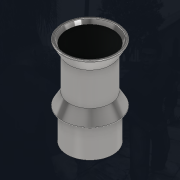
# Autodesk Inventor part: emitter
Saved by Autodesk Inventor 2021 (Build 250183000, 183)
## iProperties
Created: 2021-01-08
Part Number: emitter
Material: Generic
Document SubType Name: Modeling
Designer: Alex
Density: 1 g/cm^3
Appearance: Default
Author: Alex
Autodesk Inventor part; units mm, degrees
ref_plane "YZ Plane" through (0, 0, 0) normal (1, 0, 0) x (0, 1, 0)
ref_plane "XZ Plane" through (0, 0, 0) normal (0, 1, 0) x (-1, 0, 0)
ref_plane "XY Plane" through (0, 0, 0) normal (0, 0, 1) x (1, 0, 0)
sketch "Sketch1" plane through (0, 0, 0) normal (0, 0, 1) x (1, 0, 0)
  line L0 (0, 85.0385) -> (0, 91.0385)
  line L1 (-9, 91.0385) -> (-10, 91.0385)
  line L2 (0, 61.1) -> (0, 78.9)
  line L3 (0, 91.0385) -> (0, 96.0385)
  line L4 (-10, 91.0385) -> (-11, 91.0385)
  line L5 (-9, 91.0385) -> (-9, 85.0385)
  line L6 (-11, 91.0385) -> (-8.1132, 96.0385)
  line L7 (0, 96.0385) -> (0, 109.0385)
  line L8 (0, 96.0385) -> (0, 102.5385) construction
  line L9 (0, 102.5385) -> (-10.5, 102.5385) construction
  line L10 (-11, 114.0385) -> (-8.1132, 109.0385)
  line L11 (0, 114.0385) -> (-8, 114.0385)
  line L12 (-10, 114.0385) -> (-11, 114.0385)
  line L13 (0, 114.0385) -> (-10, 114.0385)
  line L14 (0, 109.0385) -> (0, 114.0385)
  line L15 (-8.1132, 96.0385) -> (-8.1132, 109.0385)
  line L16 (0, 0) -> (0, 114.0385)
  line L17 (0, 85.0385) -> (0, 0)
  line L18 (14, 0) -> (-14, 0)
  line L19 (0, 78.9) -> (-9, 79.0832)
  line L20 (-12, 79.0832) -> (12, 79.0832)
  line L21 (-9, 79.0832) -> (-9, 85.0385)
  point P0 (-8, 264.0385)
  point P1 (-9, 241.0385)
  point P2 (0, 79.0832)
  dimension "d0" = 6
  dimension "d1" = 10
  dimension "d2" = 5
  dimension "d3" = 9
  dimension "d4" = 13
  constraints: 44 end point, 4 symmetric about line, 3 midpoint, 2 perpendicular, 2 vertical, 1 horizontal, 1 point on line
  measures "d0" distance of L0.start L0.end
  measures "d1" distance of L0.end L1.end
  measures "d2" distance of L0.end L3.end
  measures "d3" distance of L1.start L0.end
  measures "d4" distance of L3.end L7.end
revolve "Revolution1" add sketch "Sketch1" angle 360 about axis through (0, 0, 0) along (0, 1, 0) contours L16 L20 L21 L5 L1 L4 L6 L15 L10 L12 L13 L11 L14 L7 L3 L0
sketch "Sketch2" plane through (0, 0, 0) normal (0, 0, 1) x (1, 0, 0)
  line L0 (8.1132, 109.0385) -> (11, 114.0385) construction
  line L1 (8.1132, 109.0385) -> (8.1132, 112.5385) construction
  line L2 (8.1132, 112.5385) -> (9.0002, 112.5385) construction
  line L3 (9.0002, 114.0385) -> (9.8662, 114.0385)
  line L4 (11, 114.0385) -> (-11, 114.0385) projected
  line L5 (9.8662, 114.0385) -> (9.0002, 112.5385)
  line L6 (8.1132, 109.0385) -> (-8.1132, 109.0385) projected
  line L7 (9.0002, 112.5385) -> (0, 112.5385)
  line L8 (9.0002, 114.0385) -> (0, 114.0385)
  line L9 (0, 109.0385) -> (0, 117.7347)
  point P0 (0, 0)
  point P1 (0, 112.5385)
  dimension "d6" = 3.5
  dimension "d7" = 0.887
  dimension "d8" = 1.5
  dimension "d9" = 0.866
  constraints: 14 end point, 3 point on line, 2 midpoint, 2 vertical, 1 collinear, 1 perpendicular
  measures "d6" distance of L1.start L1.end
  measures "d7" distance of L1.end L2.end
  measures "d8" distance of L2.end L3.start
  measures "d9" distance of L3.start L3.end
revolve "Revolution2" cut sketch "Sketch2" angle 360 about axis through (0, 109.0385, 0) along (0, 1, 0)
fillet "Fillet1" radius 0.3 1 edges at (11, 114.0385, 0)
fillet "Fillet2" radius 0.3 1 edges at (11, 91.0385, 0)
sketch "Sketch3" plane through (0, 79.0832, 0) normal (0, -1, 0) x (1, 0, 0)
  circle A0 centre (0, 0) radius 5
  dimension "d13" = 10
  constraints: 1 centre point, 1 coincident
  measures "d13" diameter of A0
extrude "Extrusion1" cut sketch "Sketch3" against normal blind 15
body "Solid1"
